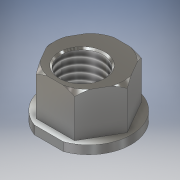
# Autodesk Inventor part: Mini Eccentric Spacer 6mm
Saved by Autodesk Inventor 2019 (Build 230136000, 136)
## iProperties
Created: 2020-11-22
Part Number: Mini Eccentric Spacer 6mm
Material: Steel
Document SubType Name: Modeling
Designer: asus
Density: 7.85 g/cm^3
Appearance: Chrome - Polished
Author: asus
Autodesk Inventor part; units mm, degrees
ref_plane "YZ Plane" through (0, 0, 0) normal (1, 0, 0) x (0, 1, 0)
ref_plane "XZ Plane" through (0, 0, 0) normal (0, 1, 0) x (-1, 0, 0)
sketch "Sketch1" plane through (0, 0, 0) normal (0, 1, 0) x (-1, 0, 0)
  arc A0 (3.8736, -1.1608) -> (1.863, 0) centre (0.9315, -3.935) ccw
  line L0 (1.863, 0) -> (0, 0)
  arc A1 (0, 0) -> (-2.0106, -1.1608) centre (0.9315, -3.935) ccw
  line L1 (-2.0106, -1.1608) -> (-2.9421, -2.7742)
  arc A2 (-2.9421, -2.7742) -> (-2.9421, -5.0958) centre (0.9315, -3.935) ccw
  line L2 (-2.9421, -5.0958) -> (-2.0106, -6.7092)
  arc A3 (-2.0106, -6.7092) -> (0, -7.87) centre (0.9315, -3.935) ccw
  line L3 (0, -7.87) -> (1.863, -7.87)
  arc A4 (1.863, -7.87) -> (3.8736, -6.7092) centre (0.9315, -3.935) ccw
  line L4 (3.8736, -6.7092) -> (4.805, -5.0958)
  arc A5 (4.805, -5.0958) -> (4.805, -2.7742) centre (0.9315, -3.935) ccw
  line L5 (4.805, -2.7742) -> (3.8736, -1.1608)
  circle A6 centre (0.9315, -3.145) radius 2.5
  line L6 (-0.7685, 0.7671) -> (2.6315, 0.7671)
  arc A7 (-0.7685, 0.7671) -> (2.6315, 0.7671) centre (0.9315, -3.935) ccw
  line L7 (-1.3404, 0) -> (-3.6123, -3.935)
  line L8 (3.2034, 0) -> (-1.3404, 0)
  line L9 (5.4752, -3.935) -> (3.2034, 0)
  line L10 (3.2034, -7.87) -> (5.4752, -3.935)
  line L11 (-1.3404, -7.87) -> (3.2034, -7.87)
  line L12 (-3.6123, -3.935) -> (-1.3404, -7.87)
  constraints: 26 end point, 14 point on circle, 8 centre point
extrude "Extrusion1" add sketch "Sketch1" against normal blind 1 contours L5 A5 L4 A4 L3 A3 L2 A2 L1 A1 L0 A0 | A0 L8 L9 | L9 L10 A5 | A1 L7 L8 | L10 L11 A4 | A2 L12 L7 | L11 L12 A3 | L6 A7
extrude "Extrusion2" add sketch "Sketch1" along normal blind 5 contours L5 A5 L4 A4 L3 A3 L2 A2 L1 A1 L0 A0 | A0 L8 L9 | L9 L10 A5 | A1 L7 L8 | L10 L11 A4 | A2 L12 L7 | L11 L12 A3
ref_plane "Work Plane1" through (1.3404, 0, -3.935) normal (0, 0, -1) x (-1, 0, 0)
sketch "Sketch2" plane through (1.3404, 0, -3.935) normal (0, 0, -1) x (-1, 0, 0)
  line L0 (0, 5) -> (-2.2719, 5) projected
  line L1 (-2.2719, 0) -> (-2.2719, 5) projected
  line L2 (-0.2281, 5) -> (4.7719, 5) projected
  line L3 (0, 5) -> (4.5437, 5) projected
  line L4 (2.2719, 5) -> (2.2719, -2.0706)
  line L5 (-2.2719, 5) -> (0, 5) projected
  line L6 (-1.7719, 5) -> (-2.2719, 4.5)
  line L7 (-2.2719, 5) -> (-2.2719, 4.5)
  line L8 (-2.2719, 5) -> (-1.7719, 5)
  point P0 (1.3404, 0)
  dimension "d7" = 0.5
  dimension "d8" = 0.5
  constraints: 8 end point, 2 point on line, 1 collinear, 1 midpoint, 1 perpendicular, 1 vertical
  measures "d7" distance from line of L6.end L0
  measures "d8" distance from line of L1 L6.start
revolve "Revolution1" cut sketch "Sketch2" angle 360 about axis through (-0.9315, 5, -3.935) along (0, -1, 0)
thread "Thread1" size "M5x0.8" class "6H" standard "ANSI Metric M Profile" full length
chamfer "Chamfer1" distance 0.2 angle 45 2 edges at (1.5685, 5, -3.145) (1.5685, -1, -3.145)
body "Solid1"
